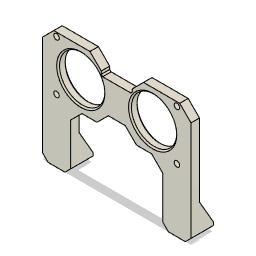
US_bracket_v18 (Autodesk Fusion 360 design; units mm, degrees)
Autodesk Fusion 360 part; units mm, degrees
sketch "Sketch1" plane through (0, 0, 0) normal (0, 0, 1) x (1, 0, 0)
  line L0 (-26.35, 10.5) -> (-26.35, -10.5)
  line L1 (-26.35, -10.5) -> (-16.35, -10.5)
  line L2 (-16.35, -10.5) -> (-16.35, 10.5)
  line L3 (-16.35, 10.5) -> (16.35, 10.5)
  line L4 (16.35, 10.5) -> (16.35, -10.5)
  line L5 (16.35, -10.5) -> (26.35, -10.5)
  line L6 (26.35, -10.5) -> (26.35, 10.5)
  line L7 (-26.35, -10.5) -> (26.35, 10.5) construction
  line L8 (-26.35, 10.5) -> (-26.35, 31)
  line L9 (-26.35, 31) -> (26.35, 31)
  line L10 (26.35, 31) -> (26.35, 10.5)
  line L11 (-22.75, 31) -> (22.75, 31) construction
  line L12 (22.75, 31) -> (22.75, 10.5) construction
  line L13 (22.75, 10.5) -> (-22.75, 10.5) construction
  line L14 (-22.75, 10.5) -> (-22.75, 31) construction
  line L15 (-22.75, 10.5) -> (22.75, 31) construction
  circle A0 centre (-21.35, 11.9) radius 0.975
  line L16 (-22.75, 20.75) -> (22.75, 20.75) construction
  line L17 (0, 10.5) -> (0, 31) construction
  circle A1 centre (-21.35, 29.6) radius 0.975
  circle A2 centre (21.35, 11.9) radius 0.975
  circle A3 centre (21.35, 29.6) radius 0.975
  circle A4 centre (-12.75, 20.75) radius 8.05
  circle A5 centre (12.75, 20.75) radius 8.05
  line L18 (0, 10.5) -> (0, 31) construction
  line L19 (5.5, 31) -> (5.5, 25.5)
  line L20 (5.5, 25.5) -> (-5.5, 25.5)
  line L21 (-5.5, 25.5) -> (-5.5, 31)
  line L22 (5, 14.5) -> (-5, 14.5)
  line L23 (-5, 14.5) -> (-5, 10.5)
  line L24 (5, 10.5) -> (5, 14.5)
  point P0 (0, 20.75)
  point P1 (0, 20.75)
  point P2 (0, 31.5)
  point P3 (0, 25.5)
  point P4 (0, 14.5)
  dimension "d3" = 10
  dimension "d4" = 52.7
  dimension "d5" = 21
  dimension "d6" = 20.5
  dimension "d7" = 45.5
  dimension "d8" = 20.5
  dimension "d9" = 1.95
  dimension "d10" = 1.4
  dimension "d11" = 1.4
  dimension "d12" = 16.1
  dimension "d13" = 10
  dimension "d16" = 11
  dimension "d17" = 5.5
  dimension "d19" = 4
  dimension "d20" = 10
  constraint perpendicular L0 L1
  constraint perpendicular L1 L2
  constraint horizontal L3
  constraint perpendicular L1 L4
  constraint vertical L6
  constraint perpendicular L4 L5
  constraint horizontal L1
  constraint equal L1 L5
  constraint equal L0 L2
  constraint equal L2 L4
  constraint equal L4 L6
  constraint midpoint origin L7
  constraint parallel L0 L8
  constraint perpendicular L8 L9
  constraint vertical L10
  constraint horizontal L11
  constraint vertical L12
  constraint horizontal L13
  constraint vertical L14
  constraint midpoint L15 P1
  constraint vertical origin P1
  constraint midpoint L14 L16.start
  constraint midpoint L12 L16.end
  constraint midpoint L13 L17.start
  constraint midpoint L9 L17.end
  constraint symmetric A0 L16 A1
  constraint symmetric A0 L17 A2
  constraint symmetric L17 A1 A3
  constraint coincident L16 A4.centre
  constraint symmetric L17 A4 A5
  constraint coincident L3 L17.start
  constraint coincident L9 L17.end
  constraint perpendicular L9 L18
  constraint midpoint L18 P1
  constraint horizontal P1 P0
  constraint vertical L19
  constraint horizontal L20
  constraint vertical L21
  constraint coincident L17 P2
  constraint coincident L9 L21.end
  constraint coincident L9 L19.start
  constraint midpoint L20 P3
  constraint coincident L18 P3
  constraint vertical L24
  constraint horizontal L22
  constraint equal L23 L24
  constraint midpoint L22 P4
  constraint coincident L18 P4
  constraint coincident L3 L23.end
  constraint coincident L3 L24.start
  measures "d3" distance of L0.end L1.end
  measures "d4" distance of L0 L6
  measures "d5" distance of L0.start L0.end
  measures "d6" distance of L0.start L8.end
  measures "d7" distance of L11.start L11.end
  measures "d8" distance of L11.start L13.end
  measures "d9" diameter of A0
  measures "d10" distance of L13 A0.centre
  measures "d11" distance of L14 A0.centre
  measures "d12" diameter of A4
  measures "d13" distance of L14 A4.centre
  measures "d16" distance of L19.end L20.end
  measures "d17" distance of L9 L20
  measures "d19" distance of L22.end L23.end
  measures "d20" distance of L22.start L22.end
extrude "Extrude1" add sketch "Sketch1" along normal blind 3 contours L0 L1 L2 L3 L4 L5 L6 L8 L9 L10 L19 L20 L21 L22 L23 L24
sketch "Sketch2" plane through (0, -10.5, 0) normal (0, -1, 0) x (1, 0, 0)
  line L0 (16.35, 0) -> (26.35, 0)
  line L1 (26.35, 0) -> (26.35, 3)
  line L2 (26.35, 3) -> (16.35, 3)
  line L3 (16.35, 3) -> (16.35, 0)
  line L4 (16.35, 0) -> (16.35, -5)
  line L5 (16.35, -5) -> (26.35, -5)
  line L6 (26.35, -5) -> (26.35, 0)
  line L7 (0, 0) -> (0, -5) construction
  line L8 (-16.35, 0) -> (-16.35, -5)
  line L9 (-16.35, -5) -> (-26.35, -5)
  line L10 (-26.35, -5) -> (-26.35, 0)
  line L11 (-26.35, 0) -> (-16.35, 0)
  circle A0 centre (21.35, -2.5) radius 1.5
  line L12 (16.35, 0) -> (26.35, -5) construction
  circle A1 centre (-21.35, -2.5) radius 1.5
  dimension "d21" = 5
  dimension "d24" = 3
  constraint coincident L0.start L3.end
  constraint perpendicular L0 L4
  constraint perpendicular L4 L5
  constraint coincident L0.end L1.start
  constraint equal L0 L5
  constraint coincident L7.start origin
  constraint vertical L7
  constraint horizontal L4.end L7.end
  constraint symmetric L0.start L7 L8.start
  constraint symmetric L4.end L7 L8.end
  constraint symmetric L5.end L7 L9.end
  constraint symmetric L0.end L7 L10.end
  constraint midpoint A0.centre L12
  constraint symmetric L7 A0 A1
  measures "d21" distance of L0 L5
  measures "d24" diameter of A0
extrude "Extrude2" add sketch "Sketch2" against normal blind 3 contours L0 L4 L5 L6 | L8 L9 L10 L11
sketch "Sketch3" plane through (26.35, 0, 0) normal (1, 0, 0) x (0, 0, -1)
  line L0 (0, -7.5) -> (0, 31)
  line L1 (0, 31) -> (-3, 31)
  line L2 (-3, 31) -> (-3, -10.5)
  line L3 (-3, -10.5) -> (5, -10.5)
  line L4 (5, -10.5) -> (5, -7.5)
  line L5 (5, -7.5) -> (0, -7.5)
  line L6 (5, -7.5) -> (0, 1.1603)
  line L7 (0, 1.1603) -> (0, -7.5)
  line L8 (5, -7.5) -> (0, -7.5)
  dimension "d27" = 60
  constraint coincident L4.end L5.start
  constraint coincident L0 L6.end
  constraint coincident L0.start L5.end
  measures "d27" angle of L5 L6
extrude "Extrude3" add sketch "Sketch3" against normal blind 1.5 contours L0 L5 L6 L7 L8
extrude "Extrude4" add sketch "Sketch3" along normal blind 1.5 from surface at -10 contours L0 L5 L6 L7 L8
extrude "Extrude5" add sketch "Sketch3" along normal blind 1.5 from surface at -52.7 contours L0 L5 L6 L7 L8
extrude "Extrude6" add sketch "Sketch3" against normal blind 1.5 from surface at -42.7 contours L0 L5 L6 L7 L8
chamfer "Chamfer1" distance 2 angle 45 8 edges at (26.35, -10.5, -1) (16.35, -10.5, -1) (-16.35, -10.5, -1) (-26.35, -10.5, -1) (-5, 14.5, 1.5) (5, 14.5, 1.5) (5, 10.5, 1.5) (-5, 10.5, 1.5)
chamfer "Chamfer1" distance 4 angle 45 4 edges at (-16.35, 10.5, 1.5) (16.35, 10.5, 1.5) (26.35, 31, 1.5) (-26.35, 31, 1.5)
chamfer "Chamfer1" distance 0.5 angle 45 6 edges at (5.2448, 23.661, 3) (5.2448, 23.661, 0) (-20.2552, 23.661, 3) (-20.2552, 23.661, 0) (-5.5, 25.5, 1.5) (5.5, 25.5, 1.5)
chamfer "Chamfer1" distance 4 angle 45 2 edges at (-5.5, 31, 1.5) (5.5, 31, 1.5)
